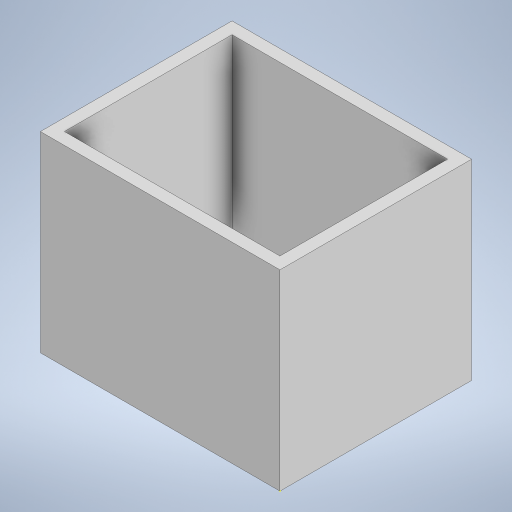
# Autodesk Inventor part: MoneyCase
Saved by Autodesk Inventor 2024 (Build 280153000, 153)
## iProperties
Created: 2025-03-28
Part Number: MoneyCase
Material: 一般
Document SubType Name: Modeling
Designer: TFG FabLab
Density: 1 g/cm^3
Appearance: 預設
Author: TFG FabLab
Autodesk Inventor part; units mm, degrees
ref_plane "YZ Plane" through (0, 0, 0) normal (1, 0, 0) x (0, 1, 0)
ref_plane "XZ Plane" through (0, 0, 0) normal (0, 1, 0) x (-1, 0, 0)
ref_plane "XY Plane" through (0, 0, 0) normal (0, 0, 1) x (1, 0, 0)
sketch "草圖1" plane through (0, 0, 0) normal (0, 1, 0) x (-1, 0, 0)
  point P0 (0, 0)
sketch "草圖2" plane through (0, 0, 0) normal (0, 1, 0) x (-1, 0, 0)
  line L0 (0, 0) -> (100, 0)
  line L1 (100, 0) -> (100, -80)
  line L2 (100, -80) -> (0, -80)
  line L3 (0, -80) -> (0, 0)
  dimension "d0" = 100
  dimension "d1" = 80
  constraints: 8 end point, 2 parallel, 1 horizontal, 1 perpendicular
  measures "d0" distance of L1.end L2.end
  measures "d1" distance of L0.end L1.end
extrude "擠出1" add sketch "草圖2" along normal blind 80
sketch "草圖3" plane through (0, 80, 0) normal (0, 1, 0) x (1, 0, 0)
  line L0 (-5, 5) -> (-95, 5)
  line L1 (-95, 5) -> (-95, 75)
  line L2 (-95, 75) -> (-5, 75)
  line L3 (-5, 75) -> (-5, 5)
  line L4 (-100, 80) -> (-100, 0) projected
  line L5 (0, 0) -> (0, 80) projected
  line L6 (-100, 0) -> (0, 0) projected
  line L7 (0, 80) -> (-100, 80) projected
  point P0 (-50, 75)
  dimension "d4" = 5
  dimension "d5" = 5
  dimension "d6" = 5
  dimension "d7" = 5
  constraints: 8 end point, 2 parallel, 1 horizontal, 1 midpoint, 1 perpendicular
  measures "d4" distance between parallel lines of L4 L1
  measures "d5" distance between parallel lines of L5 L3
  measures "d6" distance between parallel lines of L6 L0
  measures "d7" distance from line of L7 point (-50, 75)
extrude "擠出2" cut sketch "草圖3" against normal blind 75 contours L0 L1 L2 L3
